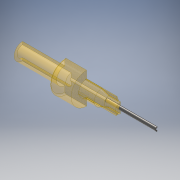
# Autodesk Inventor part: syringe_tip_14
Saved by Autodesk Inventor 2018 (Build 220112000, 112)
## iProperties
Created: 2017-11-04
Part Number: syringe_tip_14
Material: Generic
Document SubType Name: Modeling
Designer: MISAKA
Density: 1 g/cm^3
Appearance: Clear - Amber
Author: MISAKA
Autodesk Inventor part; units mm, degrees
ref_plane "YZ Plane" through (0, 0, 0) normal (1, 0, 0) x (0, 1, 0)
ref_plane "XZ Plane" through (0, 0, 0) normal (0, 1, 0) x (-1, 0, 0)
ref_plane "XY Plane" through (0, 0, 0) normal (0, 0, 1) x (1, 0, 0)
sketch "Sketch1" plane through (0, 0, 0) normal (0, 1, 0) x (-1, 0, 0)
  line L0 (37.3156, 0) -> (-29.3524, 0) projected
  line L1 (27.7916, -3) -> (12.7916, -3)
  line L2 (12.7916, -3) -> (12.7916, -5.5)
  line L3 (12.7916, -5.5) -> (5.1716, -5.5)
  line L4 (5.1716, -5.5) -> (5.1716, -2.8)
  line L5 (5.1716, -2.8) -> (-0.3284, -2.8)
  line L6 (-6.8284, -0.7) -> (-19.8284, -0.7)
  line L7 (-19.8284, -0.7) -> (-19.8284, -0.5)
  line L8 (27.7916, -3) -> (27.7916, -2)
  line L9 (27.7916, -2) -> (10.5479, -2)
  line L10 (10.5479, -2) -> (10.5479, -0.5)
  line L11 (10.5479, -0.5) -> (-2.1995, -0.5)
  line L12 (-0.3284, -2.8) -> (-2.8284, -1.8)
  line L13 (-2.8284, -1.8) -> (-6.8284, -1.8)
  line L14 (-0.3284, -2.8) -> (-5.6566, -2.8)
  line L15 (-6.8284, -1.8) -> (-6.8284, -0.7)
  line L16 (5.1716, -2.8753) -> (-5.6156, -2.8753)
  line L17 (-6.2013, -1.8) -> (-5.6156, -2.8753)
  line L18 (-6.8284, -0.7) -> (-2.1995, -0.7)
  line L19 (-2.1995, -0.7) -> (-2.1995, -0.5)
  line L20 (-2.1995, -0.5) -> (-19.8284, -0.5)
  point P0 (0, 0)
  dimension "d0" = 11
  dimension "d1" = 7.62
  dimension "d3" = 25
  dimension "d4" = 6
  dimension "d5" = 4
  dimension "d6" = 15
  dimension "d8" = 1
  dimension "d9" = 0.2
  dimension "d11" = 5.6
  dimension "d12" = 5.5
  dimension "d13" = 3.6
  dimension "d14" = 4
  dimension "d15" = 12
  constraints: 40 end point, 13 perpendicular, 4 horizontal, 3 point on line, 1 vertical
  measures "d0" diameter of L3 L0
  measures "d1" distance of L2.end L3.end
  measures "d3" distance between parallel lines of L7 L4
  measures "d4" diameter of L1 L0
  measures "d5" diameter of L9 L0
  measures "d6" distance between parallel lines of L2 L8
  measures "d8" diameter of L11 L0
  measures "d9" distance between parallel lines of L11 L6
  measures "d11" diameter of L5 L0
  measures "d12" distance from line of L4 L5.end
  measures "d13" diameter of L13 L0
  measures "d14" distance of L12.end L13.end
  measures "d15" distance between parallel lines of L15 L4
revolve "Revolution1" add sketch "Sketch1" angle 360 about axis through (-10, 0, 0) along (1, 0, 0) contours L1 L2 L3 L4 L5 L12 L13 L15 L18 L19 L11 L10 L9 L8
fillet "Fillet1" radius 0.5 1 edges at (-12.7916, 0, 5.5)
extrude "Extrusion1" add sketch "Sketch1" along normal mid plane 0.75 contours L16 L17 L14 L5 L4 | L14 L17 L13 L12
mirror "Mirror1" about plane through (0, 0, 0) normal (0, 0, 1) of "Extrusion1"
sketch "Sketch2" plane through (0, 0, 0) normal (0, 0, 1) x (1, 0, 0)
  line L0 (-5.1716, -2.8) -> (0.3284, -2.8) projected
  line L1 (-5.1716, -5.5) -> (-5.1716, 5.5) projected
  line L2 (0.3284, -2.8) -> (0.3284, -3)
  line L3 (0.3284, -3) -> (-5.1716, -3)
  line L4 (-5.1716, -3) -> (-5.1716, -1.8448)
  line L5 (-5.1716, -1.8448) -> (0.3284, -1.8448)
  line L6 (0.3284, -1.8448) -> (0.3284, -2.8)
  point P0 (0, 0)
  dimension "d18" = 0.2
  constraints: 10 end point, 3 vertical, 2 horizontal, 1 point on line
  measures "d18" distance between parallel lines of L0 L3
extrude "Extrusion2" add sketch "Sketch2" along normal mid plane 0.75
mirror "Mirror2" about plane through (0, 0, 0) normal (0, 1, 0) of "Extrusion2"
revolve "Revolution2" add sketch "Sketch1" angle 360 about axis through (-10, 0, 0) along (1, 0, 0) separate body contours L19 L18 L6 L7 L20
body "Solid1"
body "Solid2"
